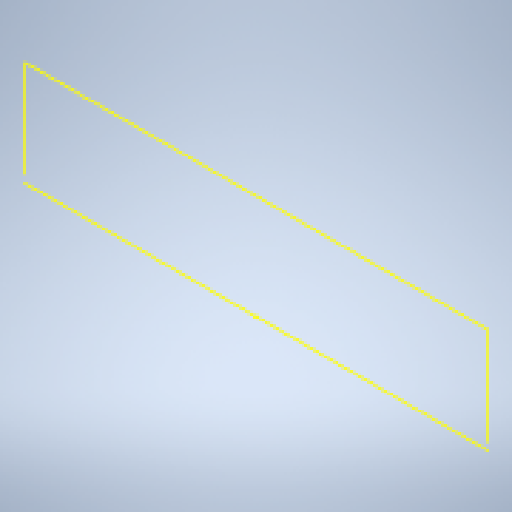
# Autodesk Inventor part: Tope
Saved by Autodesk Inventor 2024 (Build 280153000, 153)
## iProperties
Created: 2025-03-04
Part Number: Tope
Material: Genérico
Document SubType Name: Modeling
Designer: sergi
Density: 1 g/cm^3
Appearance: Valor por defecto
Author: sergi
Autodesk Inventor part; units mm, degrees
ref_plane "YZ Plane" through (0, 0, 0) normal (1, 0, 0) x (0, 1, 0)
sketch "Boceto1" plane through (0, 0, 0) normal (0, 0, 1) x (1, 0, 0)
  line L0 (-5, 2.25) -> (5, 2.25) projected
  line L1 (5, 2.25) -> (5, 0.1645) projected
  line L2 (-5, 0) -> (5, 0) projected
  line L3 (-5, 0.1645) -> (-5, 2.25) projected
  line L4 (-5, -2.25) -> (5, -2.25) projected
  line L5 (-5, 0.3078) -> (5, 0.3078) projected
  line L6 (5, 0.3078) -> (5, -2.25) projected
  line L7 (-5, 0.3078) -> (-5, -2.25) projected
  point P0 (0, 0)
extrude "Extrusión1" add sketch "Boceto1" along normal blind 10 contours L2 L6 L4 L7
sketch "Boceto2" plane through (-5, 0, 0) normal (0, 1, 0) x (1, 0, 0)
  line L0 (10, -10) -> (0, -10) projected
  line L1 (10, 0) -> (10, -10) projected
  line L2 (0, 0) -> (0, -10) projected
  line L3 (0, 0) -> (10, 0) projected
  line L4 (0, -10) -> (10, -10)
  line L5 (10, -10) -> (10, -5)
  line L6 (10, -5) -> (0, -5)
  line L7 (0, -5) -> (0, -10)
  point P0 (5, 0)
  point P1 (0, -5)
  constraints: 8 end point, 2 parallel, 1 horizontal, 1 midpoint, 1 perpendicular
ref_plane "Plano de trabajo1" through (-5, 64.15, -70) normal (0, 1, 0) x (0, 0, 1)
extrude "Extrusión2" add sketch "Boceto2" along normal up to surface (64.15 mm away) contours L0 L2 L6 L1
ref_plane "Plano de trabajo2" through (-5, -2.25, 0) normal (0, 0, 1) x (1, 0, 0)
sketch "Boceto3" plane through (5, 0, 5) normal (0, 0, -1) x (-1, 0, 0)
  line L0 (10, 64.15) -> (0, 64.15) projected
  line L1 (0, 0) -> (0, 64.15) projected
  line L2 (10, 0) -> (0, 0) projected
  line L3 (10, 0) -> (10, 64.15) projected
  line L4 (0, -2.25) -> (0, 0) projected
  line L5 (0, -2.25) -> (0, 64.15) projected
  line L6 (0, 64.15) -> (10, 64.15)
  line L7 (10, 64.15) -> (10, 61.9)
  line L8 (10, 61.9) -> (0, 61.9)
  line L9 (0, 61.9) -> (0, 64.15)
  point P0 (5, 0)
  dimension "d4" = 2.25
  constraints: 8 end point, 2 parallel, 1 horizontal, 1 perpendicular, 1 point on line
  measures "d4" distance of L6.end L7.end
extrude "Extrusión3" add sketch "Boceto3" along normal up to surface (5 mm away) contours L3 L8 L1 L0
fillet "Empalme1" radius 5 2 edges at (0, 61.9, 5) (0, 0, 5)
chamfer "Chaflán1" distance 2 angle 45 4 edges at (5, 30.95, 10) (0, -2.25, 10) (0, 64.15, 10) (-5, 30.95, 10)
